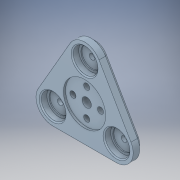
# Autodesk Inventor part: Top
Saved by Autodesk Inventor 2019.1 (Build 231200000, 200)
## iProperties
Created: 2019-01-01
Part Number: Top
Material: Generisch
Document SubType Name: Modeling
Designer: JochenAlt
Density: 1 g/cm^3
Appearance: Vorgabe
Author: JochenAlt
Autodesk Inventor part; units mm, degrees
ref_plane "YZ Plane" through (0, 0, 0) normal (1, 0, 0) x (0, 1, 0)
ref_plane "XZ Plane" through (0, 0, 0) normal (0, 1, 0) x (-1, 0, 0)
ref_plane "XY Plane" through (0, 0, 0) normal (0, 0, 1) x (1, 0, 0)
sketch "Skizze1" plane through (0, 0, 0) normal (0, 0, 1) x (1, 0, 0)
  circle A0 centre (0, 0) radius 17 construction
  circle A1 centre (0, 17) radius 5.7
  circle A2 centre (14.7224, -8.5) radius 5.7
  circle A3 centre (-14.7224, -8.5) radius 5.7
  arc A4 (6.6684, 20.85) -> (-6.6684, 20.85) centre (0, 17) ccw
  arc A5 (-21.3908, -4.65) -> (-14.7224, -16.2) centre (-14.7224, -8.5) ccw
  line L0 (6.6684, 20.85) -> (21.3908, -4.65)
  line L1 (-14.7224, -16.2) -> (14.7224, -16.2)
  line L2 (-21.3908, -4.65) -> (-6.6684, 20.85)
  arc A6 (14.7224, -16.2) -> (21.3908, -4.65) centre (14.7224, -8.5) ccw
  line L3 (0, 17) -> (14.7224, -8.5) construction
  line L4 (-14.7224, -8.5) -> (14.7224, -8.5) construction
  line L5 (-14.7224, -8.5) -> (0, 17) construction
  line L6 (-34.615, 0) -> (34.615, 0) construction
  line L7 (0, 33.265) -> (0, -26.69) construction
  circle A7 centre (0, 0) radius 9.75
  circle A8 centre (0, 17) radius 4.7
  circle A9 centre (-14.7224, -8.5) radius 4.7
  circle A10 centre (14.7224, -8.5) radius 4.7
  circle A11 centre (0, 17) radius 1.3
  circle A12 centre (-14.7224, -8.5) radius 1.3
  circle A13 centre (14.7224, -8.5) radius 1.3
  circle A14 centre (0, 0) radius 6.35 construction
  circle A15 centre (6.35, 0) radius 1.4
  circle A16 centre (0, 6.35) radius 1.4
  circle A17 centre (-6.35, 0) radius 1.4
  circle A18 centre (0, -6.35) radius 1.4
  circle A19 centre (0, 0) radius 2.15
  point P0 (0, 11.3)
  point P1 (0, 9.75)
  dimension "d1" = 11.4
  dimension "d16" = 19.5
  dimension "d17" = 12.7
  dimension "d2" = 17
  dimension "d3" = 2
  dimension "d7" = 1
  dimension "d10" = 2.6
  dimension "d20" = 360
  dimension "d22" = 2.8
  dimension "d23" = 4.3
  constraints: 17 centre point, 13 coincident, 12 end point, 9 point on circle, 7 equal radius, 6 tangent, 4 point on line, 2 equal length, 2 vertical alignment, 1 horizontal alignment, 16 other
  measures "d2" radius of A0
  measures "d10" diameter of A11
  measures "d22" diameter of A15
  measures "d23" diameter of A19
extrude "Extrusion1" add sketch "Skizze1" along normal blind 3 contours L0 A6 L1 A5 L2 A4 | A7
extrude "Extrusion2" add sketch "Skizze1" against normal blind 0.5 from surface at 0 contours A1 | A2 | A3 | L0 A6 L1 A5 L2 A4 | A7
extrude "Extrusion3" add sketch "Skizze1" against normal blind 1.5 from surface at -0.5 contours A1 | A2 | A3 | L0 A6 L1 A5 L2 A4 | A7 | A8 | A9 | A10
extrude "Extrusion5" cut sketch "Skizze1" against normal blind 1 from surface at 3 contours A7
chamfer "Fase1" distance 2 angle 45 6 edges at (0, 24.7, -2) (14.0296, 8.1, -2) (21.3908, -12.35, -2) (0, -16.2, -2) (-21.3908, -12.35, -2) (-14.0296, 8.1, -2)
chamfer "Fase2" distance 0.5 angle 45 3 edges at (-5.7, 17, 3) (-20.4224, -8.5, 3) (9.0224, -8.5, 3)
